spool_cradle_bracket (Autodesk Fusion 360 design; units mm, degrees)
part number: 2026-09-02-15-56-20-841
Autodesk Fusion 360 part; units mm, degrees
sketch "Arm triangle" plane through (0, 0, 0) normal (0, 1, 0) x (1, 0, 0)
  line L0 (0, 0) -> (0, -90)
  line L1 (0, -90) -> (150, -90)
  line L2 (150, -90) -> (0, 0)
extrude "Arm triangle (1)" add sketch "Arm triangle" along normal mid plane 24
sketch "Hook plate" plane through (0, 0, 0) normal (0, 1, 0) x (1, 0, 0)
  line L0 (0, 0) -> (6, 0)
  line L1 (6, 0) -> (6, -90)
  line L2 (6, -90) -> (0, -90)
  line L3 (0, -90) -> (0, 0)
extrude "Hook plate (1)" add sketch "Hook plate" along normal mid plane 24
sketch "Lightening cutout" plane through (0, 0, 0) normal (0, 1, 0) x (1, 0, 0)
  line L0 (14, -24.7267) -> (14, -76)
  line L1 (14, -76) -> (37.3, -76)
  line L2 (37.3, -76) -> (37.3, -38.7067)
  line L3 (37.3, -38.7067) -> (14, -24.7267)
extrude "Lightening cutout (1)" cut sketch "Lightening cutout" along normal mid plane 34
sketch "Saddle boss x=70" plane through (0, 0, 0) normal (0, 1, 0) x (1, 0, 0)
  circle A0 centre (70, -90) radius 22.7
extrude "Saddle boss x=70 (1)" add sketch "Saddle boss x=70" along normal mid plane 24
sketch "Saddle boss x=150" plane through (0, 0, 0) normal (0, 1, 0) x (1, 0, 0)
  circle A0 centre (150, -90) radius 22.7
extrude "Saddle boss x=150 (1)" add sketch "Saddle boss x=150" along normal mid plane 24
sketch "Rod pocket x=70" plane through (0, 0, 0) normal (0, 1, 0) x (1, 0, 0)
  circle A0 centre (70, -90) radius 17.1
extrude "Rod pocket x=70 (1)" cut sketch "Rod pocket x=70" along normal mid plane 34
sketch "Drop-in opening x=70" plane through (0, 0, 0) normal (0, 1, 0) x (1, 0, 0)
  line L0 (52.9, -90) -> (87.1, -90)
  line L1 (87.1, -90) -> (87.1, -117.7)
  line L2 (87.1, -117.7) -> (52.9, -117.7)
  line L3 (52.9, -117.7) -> (52.9, -90)
extrude "Drop-in opening x=70 (1)" cut sketch "Drop-in opening x=70" along normal mid plane 34
sketch "Rod pocket x=150" plane through (0, 0, 0) normal (0, 1, 0) x (1, 0, 0)
  circle A0 centre (150, -90) radius 17.1
extrude "Rod pocket x=150 (1)" cut sketch "Rod pocket x=150" along normal mid plane 34
sketch "Drop-in opening x=150" plane through (0, 0, 0) normal (0, 1, 0) x (1, 0, 0)
  line L0 (132.9, -90) -> (167.1, -90)
  line L1 (167.1, -90) -> (167.1, -117.7)
  line L2 (167.1, -117.7) -> (132.9, -117.7)
  line L3 (132.9, -117.7) -> (132.9, -90)
extrude "Drop-in opening x=150 (1)" cut sketch "Drop-in opening x=150" along normal mid plane 34
sketch "Hook profiles" plane through (0, 0, 0) normal (0, 1, 0) x (1, 0, 0)
  line L0 (0, -88) -> (-8.3, -88)
  line L1 (-8.3, -88) -> (-8.3, -71)
  line L2 (-8.3, -71) -> (-5.3, -71)
  line L3 (-5.3, -71) -> (-3.8, -72.5)
  line L4 (-3.8, -72.5) -> (-3.8, -83)
  line L5 (-3.8, -83) -> (0, -83)
  line L6 (0, -83) -> (0, -88)
  line L7 (0, -62.6) -> (-8.3, -62.6)
  line L8 (-8.3, -62.6) -> (-8.3, -45.6)
  line L9 (-8.3, -45.6) -> (-5.3, -45.6)
  line L10 (-5.3, -45.6) -> (-3.8, -47.1)
  line L11 (-3.8, -47.1) -> (-3.8, -57.6)
  line L12 (-3.8, -57.6) -> (0, -57.6)
  line L13 (0, -57.6) -> (0, -62.6)
  line L14 (0, -37.2) -> (-8.3, -37.2)
  line L15 (-8.3, -37.2) -> (-8.3, -20.2)
  line L16 (-8.3, -20.2) -> (-5.3, -20.2)
  line L17 (-5.3, -20.2) -> (-3.8, -21.7)
  line L18 (-3.8, -21.7) -> (-3.8, -32.2)
  line L19 (-3.8, -32.2) -> (0, -32.2)
  line L20 (0, -32.2) -> (0, -37.2)
  line L21 (0, -11.8) -> (-8.3, -11.8)
  line L22 (-8.3, -11.8) -> (-8.3, 5.2)
  line L23 (-8.3, 5.2) -> (-5.3, 5.2)
  line L24 (-5.3, 5.2) -> (-3.8, 3.7)
  line L25 (-3.8, 3.7) -> (-3.8, -6.8)
  line L26 (-3.8, -6.8) -> (0, -6.8)
  line L27 (0, -6.8) -> (0, -11.8)
extrude "Hook column" add sketch "Hook profiles" along normal mid plane 2.4
equation "bracketWidth = 24.0 mm" comment "drives the model; safe to edit live in Fusion"
equation "couponWidth = 8.0 mm" comment "drives the model; safe to edit live in Fusion"
equation "hookTabWidth = 2.4 mm" comment "drives the model; safe to edit live in Fusion"
equation "slotHeight = 19.05 mm" comment "reference only â edit scripts/build_rod_bracket.py and rebuild"
equation "slotPitchVertical = 25.4 mm" comment "reference only â edit scripts/build_rod_bracket.py and rebuild"
equation "slotWidth = 3.2 mm" comment "reference only â edit scripts/build_rod_bracket.py and rebuild"
equation "faceMetalThickness = 2.0 mm" comment "reference only â edit scripts/build_rod_bracket.py and rebuild"
equation "hookThroat = 3.8 mm" comment "reference only â edit scripts/build_rod_bracket.py and rebuild"
equation "hookNeckHeight = 5.0 mm" comment "reference only â edit scripts/build_rod_bracket.py and rebuild"
equation "hookLipThickness = 4.5 mm" comment "reference only â edit scripts/build_rod_bracket.py and rebuild"
equation "hookLipDrop = 12.0 mm" comment "reference only â edit scripts/build_rod_bracket.py and rebuild"
equation "plateThickness = 6.0 mm" comment "reference only â edit scripts/build_rod_bracket.py and rebuild"
equation "plateHeight = 90.0 mm" comment "reference only â edit scripts/build_rod_bracket.py and rebuild"
equation "gaugePlateThickness = 5.0 mm" comment "reference only â edit scripts/build_rod_bracket.py and rebuild"
equation "rodOuterDiameter = 33.4 mm" comment "reference only â edit scripts/build_rod_bracket.py and rebuild"
equation "saddleClearance = 0.8 mm" comment "reference only â edit scripts/build_rod_bracket.py and rebuild"
equation "saddleWall = 6.0 mm" comment "reference only â edit scripts/build_rod_bracket.py and rebuild"
equation "rearRodStandoff = 70.0 mm" comment "reference only â edit scripts/build_rod_bracket.py and rebuild"
equation "rodSpacing = 80.0 mm" comment "reference only â edit scripts/build_rod_bracket.py and rebuild"
equation "memberWidth = 14.0 mm" comment "reference only â edit scripts/build_rod_bracket.py and rebuild"
equation "hookLipChamfer = 1.5 mm" comment "reference only â edit scripts/build_rod_bracket.py and rebuild"
equation "d42 = bracketWidth"
equation "d44 = bracketWidth"
equation "d46 = bracketWidth + 10 mm"
equation "d48 = bracketWidth"
equation "d50 = bracketWidth"
equation "d52 = bracketWidth + 10 mm"
equation "d54 = bracketWidth + 10 mm"
equation "d56 = bracketWidth + 10 mm"
equation "d58 = bracketWidth + 10 mm"
equation "d60 = hookTabWidth"
named bodies: "spool_cradle_bracket"
